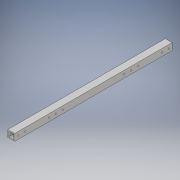
# Autodesk Inventor part: 1x1 23in
Saved by Autodesk Inventor 2018 (Build 220112000, 112)
## iProperties
Created: 2019-01-30
Part Number: 1x1 23in
Material: Generic
Document SubType Name: Modeling
Designer: s-2512711
Density: 1 g/cm^3
Appearance: Default
Author: s-2512711
Autodesk Inventor part; units mm, degrees
ref_plane "YZ Plane" through (0, 0, 0) normal (1, 0, 0) x (0, 1, 0)
ref_plane "XZ Plane" through (0, 0, 0) normal (0, 1, 0) x (-1, 0, 0)
ref_plane "XY Plane" through (0, 0, 0) normal (0, 0, 1) x (1, 0, 0)
sketch "Sketch1" plane through (0, 0, 0) normal (0, 0, 1) x (1, 0, 0)
  line L0 (0, 0) -> (25.4, 0)
  line L1 (25.4, 0) -> (25.4, 25.4)
  line L2 (25.4, 25.4) -> (0, 25.4)
  line L3 (0, 25.4) -> (0, 0)
  line L4 (3.175, 22.225) -> (22.225, 22.225)
  line L5 (22.225, 22.225) -> (22.225, 3.175)
  line L6 (22.225, 3.175) -> (3.175, 3.175)
  line L7 (3.175, 3.175) -> (3.175, 22.225)
  dimension "d0" = 25.4
  dimension "d1" = 25.4
  dimension "d2" = 3.175
  constraints: 16 end point, 4 parallel, 2 perpendicular, 1 horizontal, 3 other
  measures "d0" distance of L2.end L1.end
  measures "d1" distance of L1.end L0.end
  measures "d2" distance between parallel lines of L2 L4
extrude "Extrusion1" add sketch "Sketch1" along normal blind 584.2
sketch "Sketch2" plane through (25.4, 0, 0) normal (1, 0, 0) x (0, 0, -1)
  line L0 (0, 3.175) -> (0, 22.225) construction
  line L1 (0, 12.7) -> (-12.7, 12.7) construction
  line L2 (-12.7, 12.7) -> (-38.1, 12.7) construction
  line L3 (-584.2, 22.225) -> (-584.2, 3.175) construction
  line L4 (-584.2, 12.7) -> (-571.5, 12.7) construction
  line L5 (-571.5, 12.7) -> (-546.1, 12.7) construction
  circle A0 centre (-571.5, 12.7) radius 2.5797
  circle A1 centre (-546.1, 12.7) radius 2.5797
  circle A2 centre (-38.1, 12.7) radius 2.5797
  circle A3 centre (-12.7, 12.7) radius 2.5797
  point P0 (0, 0)
  dimension "d5" = 12.7
  dimension "d6" = 25.4
  dimension "d7" = 12.7
  dimension "d8" = 25.4
  dimension "d9" = 5.1594
  constraints: 8 end point, 4 centre point, 4 coincident, 2 horizontal, 2 midpoint, 2 point on line
  measures "d5" distance of L1.start L1.end
  measures "d6" distance of L1.end L2.end
  measures "d7" distance of L4.start L4.end
  measures "d8" distance of L4.end L5.end
  measures "d9" diameter of A0
extrude "Extrusion2" cut sketch "Sketch2" against normal blind 584.2
sketch "Sketch3" plane through (25.4, 0, 0) normal (1, 0, 0) x (0, 0, -1)
  line L0 (-584.2, 22.225) -> (-584.2, 3.175) construction
  line L1 (-584.2, 12.7) -> (-431.8, 12.7) construction
  circle A0 centre (-431.8, 12.7) radius 2.5797
  line L2 (-431.8, 12.7) -> (-457.2, 12.7) construction
  line L3 (-457.2, 12.7) -> (-406.4, 12.7) construction
  circle A1 centre (-457.2, 12.7) radius 2.5797
  circle A2 centre (-406.4, 12.7) radius 2.5797
  line L4 (0, 25.4) -> (-584.2, 25.4) construction
  line L5 (-292.1, 25.4) -> (-292.1, 0) construction
  circle A3 centre (-152.4, 12.7) radius 2.5797
  circle A4 centre (-127, 12.7) radius 2.5797
  circle A5 centre (-177.8, 12.7) radius 2.5797
  point P0 (0, 0)
  dimension "d12" = 152.4
  dimension "d13" = 5.1594
  dimension "d14" = 25.4
  dimension "d15" = 50.8
  constraints: 8 end point, 6 centre point, 3 coincident, 3 symmetric about line, 2 midpoint, 2 point on line, 1 horizontal, 1 vertical, 3 other
  measures "d12" distance of L1.start L1.end
  measures "d13" diameter of A0
  measures "d14" distance of L2.start L2.end
  measures "d15" distance of L2.end L3.end
extrude "Extrusion3" cut sketch "Sketch3" against normal blind 584.2
body "Solid1"
